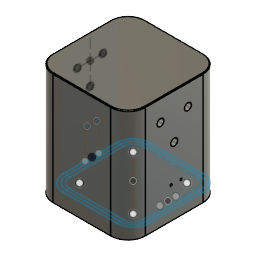
Sandwich_vis_Ar_Rés (Autodesk Fusion 360 archive; units mm, degrees)
design "Caisson_Moteur_Résine"
part number: 2026-07-29-11-15-24-907
Autodesk Fusion 360 part; units mm, degrees
sketch "Esquisse1" plane through (0, 0, 0) normal (0, 1, 0) x (1, 0, 0)
  arc A0 (59.719, 39.219) -> (44.719, 54.219) centre (44.719, 39.219) ccw construction
  line L0 (-39.219, -59.719) -> (44.719, -59.719) construction
  line L1 (-54.219, 39.219) -> (-54.219, -44.719) construction
  line L2 (-54.219, 54.219) -> (59.719, -59.719) construction
  line L3 (54.219, -12.5) -> (54.219, 12.5) construction
  arc A1 (44.719, -59.719) -> (59.719, -44.719) centre (44.719, -44.719) ccw construction
  arc A2 (-54.219, -44.719) -> (-39.219, -59.719) centre (-39.219, -44.719) ccw construction
  line L4 (44.719, 54.219) -> (-39.219, 54.219) construction
  line L5 (59.719, -44.719) -> (59.719, 39.219) construction
  arc A3 (-39.219, 54.219) -> (-54.219, 39.219) centre (-39.219, 39.219) ccw construction
  line L6 (-54.519, 39.219) -> (-54.519, -44.719)
  arc A4 (-54.519, -44.719) -> (-39.219, -60.019) centre (-39.219, -44.719) ccw
  line L7 (-39.219, -60.019) -> (44.719, -60.019)
  arc A5 (44.719, -60.019) -> (60.019, -44.719) centre (44.719, -44.719) ccw
  line L8 (60.019, -44.719) -> (60.019, 39.219)
  arc A6 (60.019, 39.219) -> (44.719, 54.519) centre (44.719, 39.219) ccw
  line L9 (44.719, 54.519) -> (-39.219, 54.519)
  arc A7 (-39.219, 54.519) -> (-54.519, 39.219) centre (-39.219, 39.219) ccw
  line L10 (-64.519, 39.219) -> (-64.519, -44.719)
  arc A8 (-64.519, -44.719) -> (-39.219, -70.019) centre (-39.219, -44.719) ccw
  line L11 (-39.219, -70.019) -> (44.719, -70.019)
  arc A9 (44.719, -70.019) -> (70.019, -44.719) centre (44.719, -44.719) ccw
  line L12 (70.019, -44.719) -> (70.019, 39.219)
  arc A10 (70.019, 39.219) -> (44.719, 64.519) centre (44.719, 39.219) ccw
  line L13 (44.719, 64.519) -> (-39.219, 64.519)
  arc A11 (-39.219, 64.519) -> (-64.519, 39.219) centre (-39.219, 39.219) ccw
  line L14 (-39.219, -65.019) -> (44.719, -65.019)
  arc A12 (44.719, -65.019) -> (65.019, -44.719) centre (44.719, -44.719) ccw
  line L15 (65.019, -44.719) -> (65.019, 39.219)
  arc A13 (65.019, 39.219) -> (44.719, 59.519) centre (44.719, 39.219) ccw
  line L16 (44.719, 59.519) -> (-39.219, 59.519)
  arc A14 (-39.219, 59.519) -> (-59.519, 39.219) centre (-39.219, 39.219) ccw
  line L17 (-59.519, 39.219) -> (-59.519, -44.719)
  arc A15 (-59.519, -44.719) -> (-39.219, -65.019) centre (-39.219, -44.719) ccw
  point P0 (54.219, 0)
  point P1 (54.219, 0)
  dimension "d2" = 15
  dimension "d3" = 15
  dimension "d4" = 113.9381
  dimension "d11" = 0.3
  dimension "d12" = 10
  dimension "d13" = 5
  constraint horizontal L4
  constraint perpendicular L1 L4
  constraint parallel L0 L4
  constraint parallel L1 L5
  constraint coincident origin L2
  constraint coincident L2.start L4
  constraint coincident L2.start L1
  constraint tangent L4 A3
  constraint tangent L1 A3
  constraint tangent A0 L4
  constraint tangent A0 L5
  constraint equal A0 A3
  constraint coincident L2.end L5
  constraint coincident L2.end L0
  constraint tangent A1 L5
  constraint tangent L0 A1
  constraint equal A1 A3
  constraint tangent L0 A2
  constraint tangent L1 A2
  constraint equal L4 L5
  constraint vertical L3
  constraint coincident P0 P1
  measures "d2" radius of A3
  measures "d3" radius of A2
  measures "d4" distance of L0 L4
extrude "Extrusion1" add sketch "Esquisse1" along normal blind 153 contours L10 A8 L11 A9 L12 A10 L13 A11 | L14 A12 L15 A13 L16 A14 L17 A15
extrude "Extrusion2" cut sketch "Esquisse1" along normal blind 2 contours L14 A12 L15 A13 L16 A14 L17 A15
sketch "Esquisse2" plane through (0, 153, 0) normal (0, 1, 0) x (-1, 0, 0)
  arc A0 (39.219, -54.519) -> (54.519, -39.219) centre (39.219, -39.219) ccw
  line L0 (39.219, -54.519) -> (-44.719, -54.519)
  arc A1 (-60.019, -39.219) -> (-44.719, -54.519) centre (-44.719, -39.219) ccw
  line L1 (-60.019, -39.219) -> (-60.019, 44.719)
  arc A2 (-44.719, 60.019) -> (-60.019, 44.719) centre (-44.719, 44.719) ccw
  line L2 (-44.719, 60.019) -> (39.219, 60.019)
  arc A3 (54.519, 44.719) -> (39.219, 60.019) centre (39.219, 44.719) ccw
  line L3 (54.519, 44.719) -> (54.519, -39.219)
  arc A4 (39.219, -64.519) -> (64.519, -39.219) centre (39.219, -39.219) ccw
  line L4 (64.519, -39.219) -> (64.519, 44.719)
  arc A5 (64.519, 44.719) -> (39.219, 70.019) centre (39.219, 44.719) ccw
  line L5 (39.219, 70.019) -> (-44.719, 70.019)
  arc A6 (-44.719, 70.019) -> (-70.019, 44.719) centre (-44.719, 44.719) ccw
  line L6 (-70.019, 44.719) -> (-70.019, -39.219)
  arc A7 (-70.019, -39.219) -> (-44.719, -64.519) centre (-44.719, -39.219) ccw
  line L7 (-44.719, -64.519) -> (39.219, -64.519)
extrude "Extrusion3" add sketch "Esquisse2" along normal blind 10 contours A0 L0 A1 L1 A2 L2 A3 L3 | A4 L4 A5 L5 A6 L6 A7 L7
fillet "Congé1" radius 2 8 edges at (-54.519, 153, 2.75) (-50.0378, 153, -50.0378) (2.75, 153, -54.519) (55.5378, 153, -50.0378) (60.019, 153, 2.75) (55.5378, 153, 55.5378) (2.75, 153, 60.019) (-50.0378, 153, 55.5378)
fillet "Congé2" radius 1 8 edges at (-64.519, 163, 2.75) (-57.1088, 163, 62.6088) (2.75, 163, 70.019) (62.6088, 163, 62.6088) (70.019, 163, 2.75) (62.6088, 163, -57.1088) (2.75, 163, -64.519) (-57.1088, 163, -57.1088)
sketch "Esquisse3" plane through (-64.519, 0, 0) normal (-1, 0, 0) x (0, 0, 1)
  line L0 (44.719, 162) -> (-39.219, 162)
  line L1 (-39.219, 162) -> (-39.219, 0)
  line L2 (-39.219, 0) -> (44.719, 0)
  line L3 (44.719, 0) -> (44.719, 162)
  line L4 (-10.75, 49) -> (10.75, 49) construction
  line L5 (10.75, 49) -> (10.75, 0) construction
  line L6 (-10.75, 0) -> (-10.75, 49) construction
  circle A0 centre (-7.25, 45.5) radius 1.55
  circle A1 centre (7.25, 45.5) radius 1.55
  line L7 (-7.25, 45.5) -> (7.25, 45.5) construction
  line L8 (2.75, 162) -> (2.75, 132) construction
  line L9 (-17.25, 132) -> (22.75, 132) construction
  circle A2 centre (22.75, 132) radius 5.1
  circle A3 centre (-17.25, 132) radius 5.1
  line L10 (2.75, 132) -> (2.75, 97.36) construction
  circle A4 centre (2.75, 97.36) radius 5.1
  point P0 (2.75, 132)
  dimension "d24" = 49
  dimension "d25" = 21.5
  dimension "d26" = 3.1
  dimension "d27" = 3.1
  dimension "d28" = 14.5
  dimension "d29" = 3.5
  dimension "d30" = 3.5
  dimension "d31" = 30
  dimension "d32" = 40
  dimension "d33" = 34.64
  dimension "d34" = 10.2
  dimension "d35" = 10.2
  dimension "d36" = 10.2
  constraint horizontal L4
  constraint vertical L5
  constraint vertical L6
  constraint horizontal L7
  constraint coincident A0.centre L7.start
  constraint coincident A1.centre L7.end
  constraint midpoint L0 L8.start
  constraint perpendicular L0 L8
  constraint horizontal L9
  constraint midpoint L9 P0
  constraint coincident P0 L8.end
  constraint coincident L9.end A2.centre
  constraint coincident L9.start A3.centre
  constraint perpendicular L9 L10
  constraint coincident L10.end A4.centre
  measures "d24" distance of L4.end L5.end
  measures "d25" distance of L4.start L4.end
  measures "d26" diameter of A1
  measures "d27" diameter of A0
  measures "d28" distance of A0.centre A1.centre
  measures "d29" distance of L4 L7
  measures "d30" distance of L6 A0.centre
  measures "d31" distance of L8.start P0
  measures "d32" distance of L9.start L9.end
  measures "d33" distance of P0 L10.end
  measures "d34" diameter of A4
  measures "d35" diameter of A3
  measures "d36" diameter of A2
extrude "Extrusion4" cut sketch "Esquisse3" against normal blind 2000 contours A0
extrude "Extrusion5" cut sketch "Esquisse3" against normal blind 2000 contours A1 | A2 | A3 | A4
scale "Echelle2" factor 1.075 about (44.719, 163, -63.519) bodies 1
equation "d4 = ( 430 mm - d2 * ( 2 * 3.141592 - 8 ) ) / 4"
equation "d33 = 0.866 * d32"
